V3D Raspberry Pi Bracket v2 (Autodesk Fusion 360 design; units mm, degrees)
Autodesk Fusion 360 part; units mm, degrees
sketch "Sketch1" plane through (0, 0, 0) normal (0, 0, 1) x (1, 0, 0)
  line L0 (29, 24.5) -> (-29, 24.5) construction
  line L1 (-29, 24.5) -> (-29, -24.5) construction
  line L2 (-29, -24.5) -> (29, -24.5) construction
  line L3 (29, -24.5) -> (29, 24.5) construction
  line L4 (29, 24.5) -> (-29, -24.5) construction
  line L5 (-29, 24.5) -> (29, -24.5) construction
  circle A0 centre (-29, 24.5) radius 0.95
  circle A1 centre (29, 24.5) radius 0.95
  circle A2 centre (29, -24.5) radius 0.95
  circle A3 centre (-29, -24.5) radius 0.95
  line L6 (-29, 24.5) -> (-29, -24.5) construction
  line L7 (29, 24.5) -> (29, -24.5) construction
  line L8 (-31.5, 8) -> (31.5, 8)
  line L9 (31.5, 8) -> (31.5, -8)
  line L10 (31.5, -8) -> (-31.5, -8)
  line L11 (-31.5, -8) -> (-31.5, 8)
  line L12 (0, 0) -> (46.2671, 0) construction
  line L13 (-23.4123, 2.75) -> (-26.5877, 2.75)
  line L14 (-26.5877, 2.75) -> (-28.1754, 0)
  line L15 (-28.1754, 0) -> (-26.5877, -2.75)
  line L16 (-26.5877, -2.75) -> (-23.4123, -2.75)
  line L17 (-23.4123, -2.75) -> (-21.8246, 0)
  line L18 (-21.8246, 0) -> (-23.4123, 2.75)
  circle A4 centre (-25, 0) radius 1.75
  line L19 (0, 0) -> (0, 20.3309) construction
  line L20 (28.1754, 0) -> (26.5877, -2.75)
  line L21 (26.5877, -2.75) -> (23.4123, -2.75)
  line L22 (23.4123, -2.75) -> (21.8246, 0)
  line L23 (21.8246, 0) -> (23.4123, 2.75)
  line L24 (23.4123, 2.75) -> (26.5877, 2.75)
  line L25 (26.5877, 2.75) -> (28.1754, 0)
  circle A5 centre (25, 0) radius 1.75
  line L26 (17.5, 5.5) -> (-17.5, 5.5)
  line L27 (-17.5, 5.5) -> (-17.5, -5.5)
  line L28 (-17.5, -5.5) -> (17.5, -5.5)
  line L29 (17.5, -5.5) -> (17.5, 5.5)
  line L30 (17.5, 5.5) -> (-17.5, -5.5) construction
  line L31 (-17.5, 5.5) -> (17.5, -5.5) construction
  line L32 (-29, 27.3868) -> (-31.5, 25.9434)
  line L33 (-31.5, 25.9434) -> (-31.5, 23.0566)
  line L34 (-31.5, 23.0566) -> (-29, 21.6132)
  line L35 (-29, 21.6132) -> (-26.5, 23.0566)
  line L36 (-26.5, 23.0566) -> (-26.5, 25.9434)
  line L37 (-26.5, 25.9434) -> (-29, 27.3868)
  line L38 (-26.5, -25.9434) -> (-26.5, -23.0566)
  line L39 (-26.5, -23.0566) -> (-29, -21.6132)
  line L40 (-29, -21.6132) -> (-31.5, -23.0566)
  line L41 (-31.5, -23.0566) -> (-31.5, -25.9434)
  line L42 (-31.5, -25.9434) -> (-29, -27.3868)
  line L43 (-29, -27.3868) -> (-26.5, -25.9434)
  line L44 (31.5, -25.9434) -> (31.5, -23.0566)
  line L45 (31.5, -23.0566) -> (29, -21.6132)
  line L46 (29, -21.6132) -> (26.5, -23.0566)
  line L47 (26.5, -23.0566) -> (26.5, -25.9434)
  line L48 (26.5, -25.9434) -> (29, -27.3868)
  line L49 (29, -27.3868) -> (31.5, -25.9434)
  line L50 (29, 27.3868) -> (26.5, 25.9434)
  line L51 (26.5, 25.9434) -> (26.5, 23.0566)
  line L52 (26.5, 23.0566) -> (29, 21.6132)
  line L53 (29, 21.6132) -> (31.5, 23.0566)
  line L54 (31.5, 23.0566) -> (31.5, 25.9434)
  line L55 (31.5, 25.9434) -> (29, 27.3868)
  line L56 (-31.5, 23.0566) -> (-26.5, 23.0566)
  line L57 (-26.5, 23.0566) -> (-26.5, -23.0566)
  line L58 (-26.5, -23.0566) -> (-31.5, -23.0566)
  line L59 (-31.5, -23.0566) -> (-31.5, 23.0566)
  line L60 (26.5, 23.0566) -> (31.5, 23.0566)
  line L61 (31.5, 23.0566) -> (31.5, -23.0566)
  line L62 (31.5, -23.0566) -> (26.5, -23.0566)
  line L63 (26.5, -23.0566) -> (26.5, 23.0566)
  point P0 (-25, 0)
  point P1 (-29, 24.5)
  point P2 (-29, -24.5)
  point P3 (29, -24.5)
  point P4 (29, 24.5)
  dimension "d1" = 58
  dimension "d2" = 49
  dimension "d3" = 1.9
  dimension "d5" = 16
  dimension "d7" = 5.5
  dimension "d8" = 3.5
  dimension "d9" = 50
  dimension "d16" = 11
  dimension "d17" = 35
  dimension "d20" = 5
  constraint horizontal L0
  constraint perpendicular L0 L1
  constraint parallel L0 L2
  constraint parallel L1 L3
  constraint coincident L4 L12.start
  constraint coincident L5 L12.start
  constraint coincident L12.start L19.start
  constraint coincident P1 L0.end
  constraint coincident P4 L0.start
  constraint coincident P3 L2.end
  constraint coincident P2 L1.end
  constraint equal A2 A3
  constraint equal A1 A2
  constraint equal A0 A1
  constraint perpendicular L2 L6
  constraint perpendicular L2 L7
  constraint horizontal L8
  constraint vertical L9
  constraint horizontal L10
  constraint vertical L11
  constraint symmetric L8 L10 L12
  constraint horizontal L13
  constraint coincident P0 A4.centre
  constraint perpendicular L12 L19
  constraint symmetric L13.start L19 L23.end
  constraint symmetric L13.end L19 L24.end
  constraint symmetric L14.end L19 L20.start
  constraint symmetric L15.end L19 L20.end
  constraint symmetric L16.end L19 L21.end
  constraint symmetric L17.end L19 L22.end
  constraint symmetric A4 L19 A5
  constraint coincident L12 P0
  constraint horizontal L26
  constraint perpendicular L26 L27
  constraint parallel L26 L28
  constraint parallel L27 L29
  constraint coincident L30 L12.start
  constraint coincident L31 L12.start
  constraint equal L32 L50
  constraint equal L32 L40
  constraint equal L40 L45
  constraint vertical L54
  constraint vertical L44
  constraint vertical L38
  constraint vertical L36
  constraint horizontal L56
  constraint vertical L57
  constraint horizontal L58
  constraint vertical L59
  constraint horizontal L60
  constraint vertical L61
  constraint horizontal L62
  constraint vertical L63
  measures "d1" distance of P2 L2.end
  measures "d2" distance of P1 L1.end
  measures "d3" diameter of A0
  measures "d5" distance of L8 L10
  measures "d7" distance of L13 L16
  measures "d8" diameter of A4
  measures "d9" distance of P0 A5.centre
  measures "d16" distance of L26.start L28.end
  measures "d17" distance of L26.start L26.end
  measures "d20" distance of L50 L53
extrude "Extrude1" add sketch "Sketch1" along normal blind 6 contours A0 | A1 | A2 | A3 | L8 L34 L35 L57 L59 | L8 L10 L11 L13 L14 L15 L16 L57 L59 | L8 L10 L13 L16 L17 L18 L21 L22 L23 L24 L57 L63 | L10 L39 L40 L57 L59 | L34 L35 L56 | L32 L33 L36 L37 L56 | L8 L52 L53 L61 L63 | L8 L9 L10 L20 L21 L24 L25 L61 L63 | L13 L14 L15 L16 A4 L57 | L13 L16 L17 L18 A4 L57 | L38 L41 L42 L43 L58 | L39 L40 L58 | L21 L22 L23 L24 A5 L63 | L20 L21 L24 L25 A5 L63 | L52 L53 L60 | L50 L51 L54 L55 L60 | L10 L45 L46 L61 L63 | L44 L47 L48 L49 L62 | L45 L46 L62
extrude "Extrude2" add sketch "Sketch1" along normal blind 3 draft -10 from surface at 6 contours A0 | A1 | A2 | A3 | L34 L35 L56 | L32 L33 L36 L37 L56 | L38 L41 L42 L43 L58 | L39 L40 L58 | L52 L53 L60 | L50 L51 L54 L55 L60 | L44 L47 L48 L49 L62 | L45 L46 L62
extrude "Extrude4" cut sketch "Sketch1" along normal through all contours A0 | A1 | A2 | A3
extrude "Extrude3" cut sketch "Sketch1" along normal through all from surface at 1.2 contours L13 L14 L15 L16 A4 L57 | L13 L16 L17 L18 A4 L57 | L21 L22 L23 L24 A5 L63 | L20 L21 L24 L25 A5 L63
chamfer "Chamfer1" distance 4 angle 45 8 edges at (-17.5, 5.5, 3) (-17.5, -5.5, 3) (17.5, -5.5, 3) (17.5, 5.5, 3) (-26.5, -8, 3) (-26.5, 8, 3) (26.5, 8, 3) (26.5, -8, 3)
chamfer "Chamfer2" distance 2 angle 45 4 edges at (0, 8, 6) (0, -8, 6) (31.5, 0, 6) (-31.5, 0, 6)
